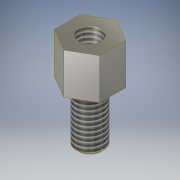
# Autodesk Inventor part: standoff (1466814)
Saved by Autodesk Inventor 2017 (Build 210142000, 142)
## iProperties
Part Number: standoff (1466814)
Material: Generisch
Document SubType Name: Modeling
Designer: ExCISS
Density: 1 g/cm^3
Appearance: Nickel
Author: ExCISS
Autodesk Inventor part; units mm, degrees
ref_plane "YZ Plane" through (0, 0, 0) normal (1, 0, 0) x (0, 1, 0)
ref_plane "XZ Plane" through (0, 0, 0) normal (0, 1, 0) x (-1, 0, 0)
ref_plane "XY Plane" through (0, 0, 0) normal (0, 0, 1) x (1, 0, 0)
sketch "Skizze1" plane through (0, 0, 0) normal (0, 0, 1) x (1, 0, 0)
  line L0 (-2.5, 1.4434) -> (0, 2.8868)
  line L1 (0, 2.8868) -> (2.5, 1.4434)
  line L2 (2.5, 1.4434) -> (2.5, -1.4434)
  line L3 (2.5, -1.4434) -> (0, -2.8868)
  line L4 (0, -2.8868) -> (-2.5, -1.4434)
  line L5 (-2.5, -1.4434) -> (-2.5, 1.4434)
  point P0 (0, 0)
  point P1 (0, 0)
  point P2 (0, 0)
  dimension "d2" = 5
  constraints: 12 end point, 2 coincident, 1 vertical, 13 other
  measures "d2" distance between parallel lines of L2 L5
extrude "Extrusion1" add sketch "Skizze1" along normal mid plane 4.5
sketch "Skizze3" plane through (0, 0, 2.25) normal (0, 0, 1) x (1, 0, 0)
  point P0 (0, 0)
  point P1 (0, 0)
  constraints: 1 coincident
hole "Bohrung1" at (0, 0, 2.25) direction (0, 0, -1) diameter 2.459 depth 8.8 tip angle 118 thread size "M3x0.5" class "6H" standard "ISO Metric profile"
sketch "Skizze4" plane through (0, 0, -2.25) normal (0, 0, -1) x (-1, 0, 0)
  circle A0 centre (0, 0) radius 1.5
  dimension "d17" = 3
  constraints: 1 centre point, 1 coincident
  measures "d17" diameter of A0
extrude "Extrusion3" add sketch "Skizze4" along normal blind 6
thread "Gewinde2" size "M3x0.5" class "6g" standard "ISO Metric profile" full length
chamfer "Fase1" distance 0.25 angle 45 1 edges at (1.5, 0, -8.25)
